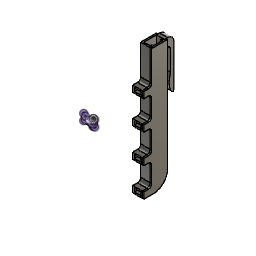
WaterLevelSensor (Autodesk Fusion 360 design; units mm, degrees)
Autodesk Fusion 360 part; units mm, degrees
note: some values were not read from the file. Set by a fixed rule: which sketch regions a step uses.
sketch "Sketch1" plane through (0, 0, 0) normal (1, 0, 0) x (0, 1, 0)
  line L0 (0, 200) -> (10, 200)
  line L1 (10, 200) -> (10, 129)
  line L2 (1, 120) -> (0, 120)
  line L3 (0, 120) -> (-5, 120)
  line L4 (-5, 120) -> (-5, 124)
  line L5 (-5, 124) -> (-2, 124)
  line L6 (-5, 142.3333) -> (-2, 142.3333)
  line L7 (-5, 138.3333) -> (-5, 142.3333)
  line L8 (-2, 138.3333) -> (-5, 138.3333)
  line L9 (-5, 160.6667) -> (-2, 160.6667)
  line L10 (-5, 156.6667) -> (-5, 160.6667)
  line L11 (-2, 156.6667) -> (-5, 156.6667)
  line L12 (-5, 179) -> (-2, 179)
  line L13 (-5, 175) -> (-5, 179)
  line L14 (-2, 175) -> (-5, 175)
  line L15 (0, 181) -> (0, 200)
  line L16 (0, 162.6667) -> (0, 173)
  line L17 (0, 126) -> (0, 136.3333)
  line L18 (0, 144.3333) -> (0, 154.6667)
  arc A0 (1, 120) -> (10, 129) centre (1, 129) ccw
  arc A1 (-2, 179) -> (0, 181) centre (-2, 181) ccw
  arc A2 (0, 173) -> (-2, 175) centre (-2, 173) ccw
  arc A3 (-2, 160.6667) -> (0, 162.6667) centre (-2, 162.6667) ccw
  arc A4 (0, 154.6667) -> (-2, 156.6667) centre (-2, 154.6667) ccw
  arc A5 (-2, 142.3333) -> (0, 144.3333) centre (-2, 144.3333) ccw
  arc A6 (0, 136.3333) -> (-2, 138.3333) centre (-2, 136.3333) ccw
  arc A7 (-2, 124) -> (0, 126) centre (-2, 126) ccw
  line L19 (0, 121) -> (-5, 121)
  line L20 (-5, 123) -> (-2, 123)
  arc A8 (-2, 123) -> (1, 126) centre (-2, 126) ccw
  line L21 (1, 126) -> (1, 136.3333)
  arc A9 (1, 136.3333) -> (-2, 139.3333) centre (-2, 136.3333) ccw
  line L22 (-2, 139.3333) -> (-5, 139.3333)
  line L23 (-5, 141.3333) -> (-2, 141.3333)
  arc A10 (-2, 141.3333) -> (1, 144.3333) centre (-2, 144.3333) ccw
  line L24 (1, 144.3333) -> (1, 154.6667)
  arc A11 (1, 154.6667) -> (-2, 157.6667) centre (-2, 154.6667) ccw
  line L25 (-2, 157.6667) -> (-5, 157.6667)
  line L26 (-5, 159.6667) -> (-2, 159.6667)
  arc A12 (-2, 159.6667) -> (1, 162.6667) centre (-2, 162.6667) ccw
  line L27 (1, 162.6667) -> (1, 173)
  arc A13 (1, 173) -> (-2, 176) centre (-2, 173) ccw
  line L28 (-2, 176) -> (-5, 176)
  line L29 (-5, 178) -> (-2, 178)
  arc A14 (-2, 178) -> (1, 181) centre (-2, 181) ccw
  line L30 (1, 181) -> (1, 200)
  line L31 (9, 200) -> (9, 129)
  arc A15 (1, 121) -> (9, 129) centre (1, 129) ccw
  line L32 (1, 121) -> (0, 121)
  line L33 (10, 200) -> (11, 200)
  line L34 (15, 196) -> (15, 170)
  line L35 (13, 180) -> (13, 193)
  line L36 (11, 195) -> (10, 195)
  spline S0 degree 5 poles (13, 180) (12.9242, 179.8) (12.7791, 179.4) (12.5813, 178.8) (12.3581, 178) (12.1509, 177) (12.0221, 176) (11.978, 175) (12.0221, 174) (12.1509, 173) (12.3581, 172) (12.5813, 171.2) (12.7791, 170.6) (12.9242, 170.2) (13, 170) knots 0 0 0 0 0 0 0.1 0.2 0.3 0.4 0.5 0.6 0.7 0.8 0.9 1 1 1 1 1 1
  arc A16 (15, 196) -> (11, 200) centre (11, 196) ccw
  arc A17 (13, 193) -> (11, 195) centre (11, 193) ccw
  spline S1 degree 5 poles (13, 170) (13.0376, 169.953) (13.1131, 169.8604) (13.227, 169.726) (13.38, 169.5556) (13.5735, 169.3586) (13.7694, 169.179) (13.9418, 169.0396) (14.076, 168.9434) (14.1707, 168.8813) (14.2252, 168.8475) (14.2391, 168.8391) knots 0 0 0 0 0 0 0.1 0.2 0.3 0.4 0.5 0.6 0.634052 0.634052 0.634052 0.634052 0.634052 0.634052
  line L37 (15, 170) -> (15, 169.2656)
  arc A18 (14.2391, 168.8391) -> (15, 169.2656) centre (14.5, 169.2656) ccw
  point P0 (0, 124)
  point P1 (12, 175)
  point P2 (14, 169)
  dimension "d1" = 10
  dimension "d2" = 80
  dimension "d3" = 5
  dimension "d4" = 4
  dimension "d10" = 9
  dimension "d11" = 2
  dimension "d12" = 4
  dimension "d13" = 2
  dimension "d14" = 0.5
  constraint horizontal L0
  constraint vertical L1
  constraint horizontal L2
  constraint vertical L17
  constraint horizontal L3
  constraint vertical L4
  constraint horizontal L5
  constraint collinear L15 L17
  constraint collinear L16 L17
  constraint collinear L17 L18
  constraint tangent L1 A0
  constraint tangent L2 A0
  constraint tangent L12 A1
  constraint tangent L15 A1
  constraint tangent L14 A2
  constraint tangent L16 A2
  constraint equal A1 A2
  constraint tangent L9 A3
  constraint tangent L16 A3
  constraint equal A1 A3
  constraint tangent L11 A4
  constraint tangent L18 A4
  constraint equal A1 A4
  constraint tangent L6 A5
  constraint tangent L18 A5
  constraint equal A1 A5
  constraint tangent L8 A6
  constraint tangent L17 A6
  constraint equal A1 A6
  constraint coincident P0 L5
  constraint coincident P0 L17
  constraint tangent L5 A7
  constraint tangent L17 A7
  constraint equal A1 A7
  constraint concentric A7 A8
  constraint concentric A6 A9
  constraint concentric A5 A10
  constraint concentric A4 A11
  constraint concentric A3 A12
  constraint concentric A2 A13
  constraint concentric A1 A14
  constraint concentric A0 A15
  constraint tangent L21 A9
  constraint tangent A9 L22
  constraint tangent A11 L25
  constraint tangent L20 A8
  constraint tangent L31 A15
  constraint tangent A8 L21
  constraint tangent L23 A10
  constraint tangent A10 L24
  constraint tangent L24 A11
  constraint tangent L27 A13
  constraint tangent L26 A12
  constraint tangent A12 L27
  constraint tangent A13 L28
  constraint tangent L29 A14
  constraint tangent A14 L30
  constraint tangent A15 L32
  constraint coincident L4 L20.start
  constraint coincident L4 L19.end
  constraint coincident L0 L31.start
  constraint coincident L0 L30.end
  constraint perpendicular L1 L33
  constraint perpendicular L33 L34
  constraint coincident L1 L36.end
  constraint perpendicular L1 L36
  constraint tangent L33 A16
  constraint tangent L34 A16
  constraint tangent L35 A17
  constraint tangent L36 A17
  constraint tangent S1 A18
  constraint tangent L37 A18
  measures "d1" distance of L0.start L0.end
  measures "d2" distance of L0.start L2.end
  measures "d3" distance of L2.end L3.end
  measures "d4" distance of L2.end P0
  measures "d10" radius of A0
  measures "d11" radius of A1
  measures "d12" radius of A16
  measures "d13" radius of A17
  measures "d14" radius of A18
extrude "Extrude1" add sketch "Sketch1" along normal blind 1 makes body 1
extrude "Extrude2" add sketch "Sketch1" along normal blind 6 contours L0 L12 L13 L15 A1 L29 A14 L30 | L0 L1 L2 L3 L4 A0 L19 L31 A15 L32 | L1 L33 L34 L35 L36 S0 A16 A17 S1 L37 A18 | L9 L10 L13 L14 L16 A2 A3 L26 A12 L27 A13 L28 | L4 L5 L7 L8 L17 A6 A7 L20 A8 L21 A9 L22 | L6 L7 L10 L11 L18 A4 A5 L23 A10 L24 A11 L25 bodies 1
extrude "Extrude3" cut sketch "Sketch1" along normal blind 1 contours L1 L33 L34 L35 L36 S0 A16 A17 S1 L37 A18 bodies 1
sketch "Sketch2" plane through (6, 0, 0) normal (1, 0, 0) x (0, 1, 0)
  spline S0 degree 5 poles (13, 180) (12.9242, 179.8) (12.7791, 179.4) (12.5813, 178.8) (12.3581, 178) (12.1509, 177) (12.0221, 176) (11.978, 175) (12.0221, 174) (12.1509, 173) (12.3581, 172) (12.5813, 171.2) (12.7791, 170.6) (12.9242, 170.2) (13, 170) knots 0 0 0 0 0 0 0.1 0.2 0.3 0.4 0.5 0.6 0.7 0.8 0.9 1 1 1 1 1 1
  spline S1 degree 5 poles (13, 170) (13.0376, 169.953) (13.1131, 169.8604) (13.227, 169.726) (13.38, 169.5556) (13.5735, 169.3586) (13.7694, 169.179) (13.9418, 169.0396) (14.076, 168.9434) (14.1707, 168.8813) (14.2252, 168.8475) (14.2391, 168.8391) knots 0 0 0 0 0 0 0.1 0.2 0.3 0.4 0.5 0.6 0.634052 0.634052 0.634052 0.634052 0.634052 0.634052
  arc A0 (14.2391, 168.8391) -> (15, 169.2656) centre (14.5, 169.2656) ccw
  line L0 (15, 169.2656) -> (15, 196)
  arc A1 (15, 196) -> (11, 200) centre (11, 196) ccw
  line L1 (11, 200) -> (9, 200)
  line L2 (9, 200) -> (9, 129)
  arc A2 (1, 121) -> (9, 129) centre (1, 129) ccw
  line L3 (1, 121) -> (-5, 121)
  line L4 (-5, 121) -> (-5, 120)
  line L5 (-5, 120) -> (1, 120)
  arc A3 (1, 120) -> (10, 129) centre (1, 129) ccw
  line L6 (10, 129) -> (10, 195)
  line L7 (10, 195) -> (11, 195)
  arc A4 (13, 193) -> (11, 195) centre (11, 193) ccw
  line L8 (13, 193) -> (13, 180)
  line L9 (-5, 178) -> (-2, 178)
  arc A5 (-2, 178) -> (1, 181) centre (-2, 181) ccw
  line L10 (1, 181) -> (1, 200)
  line L11 (1, 200) -> (0, 200)
  line L12 (0, 200) -> (0, 181)
  arc A6 (-2, 179) -> (0, 181) centre (-2, 181) ccw
  line L13 (-2, 179) -> (-5, 179)
  line L14 (-5, 179) -> (-5, 178)
  line L15 (-5, 159.6667) -> (-2, 159.6667)
  arc A7 (-2, 159.6667) -> (1, 162.6667) centre (-2, 162.6667) ccw
  line L16 (1, 162.6667) -> (1, 173)
  arc A8 (1, 173) -> (-2, 176) centre (-2, 173) ccw
  line L17 (-2, 176) -> (-5, 176)
  line L18 (-5, 176) -> (-5, 175)
  line L19 (-5, 175) -> (-2, 175)
  arc A9 (0, 173) -> (-2, 175) centre (-2, 173) ccw
  line L20 (0, 173) -> (0, 162.6667)
  arc A10 (-2, 160.6667) -> (0, 162.6667) centre (-2, 162.6667) ccw
  line L21 (-2, 160.6667) -> (-5, 160.6667)
  line L22 (-5, 160.6667) -> (-5, 159.6667)
  line L23 (-5, 141.3333) -> (-2, 141.3333)
  arc A11 (-2, 141.3333) -> (1, 144.3333) centre (-2, 144.3333) ccw
  line L24 (1, 144.3333) -> (1, 154.6667)
  arc A12 (1, 154.6667) -> (-2, 157.6667) centre (-2, 154.6667) ccw
  line L25 (-2, 157.6667) -> (-5, 157.6667)
  line L26 (-5, 157.6667) -> (-5, 156.6667)
  line L27 (-5, 156.6667) -> (-2, 156.6667)
  arc A13 (0, 154.6667) -> (-2, 156.6667) centre (-2, 154.6667) ccw
  line L28 (0, 154.6667) -> (0, 144.3333)
  arc A14 (-2, 142.3333) -> (0, 144.3333) centre (-2, 144.3333) ccw
  line L29 (-2, 142.3333) -> (-5, 142.3333)
  line L30 (-5, 142.3333) -> (-5, 141.3333)
  line L31 (-5, 123) -> (-2, 123)
  arc A15 (-2, 123) -> (1, 126) centre (-2, 126) ccw
  line L32 (1, 126) -> (1, 136.3333)
  arc A16 (1, 136.3333) -> (-2, 139.3333) centre (-2, 136.3333) ccw
  line L33 (-2, 139.3333) -> (-5, 139.3333)
  line L34 (-5, 139.3333) -> (-5, 138.3333)
  line L35 (-5, 138.3333) -> (-2, 138.3333)
  arc A17 (0, 136.3333) -> (-2, 138.3333) centre (-2, 136.3333) ccw
  line L36 (0, 136.3333) -> (0, 126)
  arc A18 (-2, 124) -> (0, 126) centre (-2, 126) ccw
  line L37 (-2, 124) -> (-5, 124)
  line L38 (-5, 124) -> (-5, 123)
  line L39 (-5, 139.3333) -> (-2, 139.3333)
  arc A19 (1, 136.3333) -> (-2, 139.3333) centre (-2, 136.3333) ccw
  line L40 (1, 136.3333) -> (1, 126)
  arc A20 (-2, 123) -> (1, 126) centre (-2, 126) ccw
  line L41 (-2, 123) -> (-5, 123)
  line L42 (-5, 123) -> (-5, 121)
  line L43 (-5, 121) -> (1, 121)
  arc A21 (1, 121) -> (9, 129) centre (1, 129) ccw
  line L44 (9, 129) -> (9, 200)
  line L45 (9, 200) -> (1, 200)
  line L46 (1, 200) -> (1, 181)
  arc A22 (-2, 178) -> (1, 181) centre (-2, 181) ccw
  line L47 (-2, 178) -> (-5, 178)
  line L48 (-5, 178) -> (-5, 176)
  line L49 (-5, 176) -> (-2, 176)
  arc A23 (1, 173) -> (-2, 176) centre (-2, 173) ccw
  line L50 (1, 173) -> (1, 162.6667)
  arc A24 (-2, 159.6667) -> (1, 162.6667) centre (-2, 162.6667) ccw
  line L51 (-2, 159.6667) -> (-5, 159.6667)
  line L52 (-5, 159.6667) -> (-5, 157.6667)
  line L53 (-5, 157.6667) -> (-2, 157.6667)
  arc A25 (1, 154.6667) -> (-2, 157.6667) centre (-2, 154.6667) ccw
  line L54 (1, 154.6667) -> (1, 144.3333)
  arc A26 (-2, 141.3333) -> (1, 144.3333) centre (-2, 144.3333) ccw
  line L55 (-2, 141.3333) -> (-5, 141.3333)
  line L56 (-5, 141.3333) -> (-5, 139.3333)
  line L57 (10, 195) -> (10, 200)
  line L58 (1.2, 200) -> (1.2, 181)
  arc A27 (-2, 177.8) -> (1.2, 181) centre (-2, 181) ccw
  line L59 (-2, 177.8) -> (-4.8, 177.8)
  line L60 (-4.8, 177.8) -> (-4.8, 176.2)
  line L61 (-4.8, 176.2) -> (-2, 176.2)
  arc A28 (1.2, 173) -> (-2, 176.2) centre (-2, 173) ccw
  line L62 (1.2, 173) -> (1.2, 162.6667)
  arc A29 (-2, 159.4667) -> (1.2, 162.6667) centre (-2, 162.6667) ccw
  line L63 (-2, 159.4667) -> (-4.8, 159.4667)
  line L64 (-4.8, 159.4667) -> (-4.8, 157.8667)
  line L65 (-4.8, 157.8667) -> (-2, 157.8667)
  arc A30 (1.2, 154.6667) -> (-2, 157.8667) centre (-2, 154.6667) ccw
  line L66 (1.2, 154.6667) -> (1.2, 144.3333)
  arc A31 (-2, 141.1333) -> (1.2, 144.3333) centre (-2, 144.3333) ccw
  line L67 (-2, 141.1333) -> (-4.8, 141.1333)
  line L68 (-4.8, 141.1333) -> (-4.8, 139.5333)
  line L69 (-4.8, 139.5333) -> (-2, 139.5333)
  arc A32 (1.2, 136.3333) -> (-2, 139.5333) centre (-2, 136.3333) ccw
  line L70 (1.2, 136.3333) -> (1.2, 126)
  arc A33 (-2, 122.8) -> (1.2, 126) centre (-2, 126) ccw
  line L71 (-2, 122.8) -> (-4.8, 122.8)
  line L72 (-4.8, 122.8) -> (-4.8, 121.2)
  line L73 (-4.8, 121.2) -> (1, 121.2)
  arc A34 (1, 121.2) -> (8.8, 129) centre (1, 129) ccw
  line L74 (8.8, 129) -> (8.8, 200)
  arc A35 (-0.7194, 177) -> (2.2, 181) centre (-2, 181) ccw
  line L75 (2.2, 200) -> (2.2, 181)
  line L76 (7.8, 129) -> (7.8, 200)
  arc A36 (1, 122.2) -> (7.8, 129) centre (1, 129) ccw
  line L77 (-0.2111, 122.2) -> (1, 122.2)
  arc A37 (-0.2111, 122.2) -> (2.2, 126) centre (-2, 126) ccw
  line L78 (2.2, 136.3333) -> (2.2, 126)
  arc A38 (2.2, 136.3333) -> (-0.7194, 140.3333) centre (-2, 136.3333) ccw
  arc A39 (-0.7194, 140.3333) -> (2.2, 144.3333) centre (-2, 144.3333) ccw
  line L79 (2.2, 154.6667) -> (2.2, 144.3333)
  arc A40 (2.2, 154.6667) -> (-0.7194, 158.6667) centre (-2, 154.6667) ccw
  arc A41 (-0.7194, 158.6667) -> (2.2, 162.6667) centre (-2, 162.6667) ccw
  line L80 (2.2, 173) -> (2.2, 162.6667)
  arc A42 (2.2, 173) -> (-0.7194, 177) centre (-2, 173) ccw
  constraint coincident L6.end L7.start
  constraint midpoint L1 L57.end
  constraint concentric A22 A27
  constraint concentric A23 A28
  constraint concentric A24 A29
  constraint concentric A25 A30
  constraint concentric A26 A31
  constraint concentric A19 A32
  constraint concentric A20 A33
  constraint concentric A21 A34
  constraint tangent L62 A29
  constraint tangent L61 A28
  constraint tangent A28 L62
  constraint tangent L58 A27
  constraint tangent A27 L59
  constraint tangent A29 L63
  constraint tangent L65 A30
  constraint tangent A30 L66
  constraint tangent L66 A31
  constraint tangent A31 L67
  constraint tangent L69 A32
  constraint tangent A32 L70
  constraint tangent L70 A33
  constraint tangent A33 L71
  constraint tangent L73 A34
  constraint tangent A34 L74
  constraint concentric A22 A35
  constraint concentric A21 A36
  constraint concentric A20 A37
  constraint concentric A19 A38
  constraint concentric A26 A39
  constraint concentric A25 A40
  constraint concentric A24 A41
  constraint concentric A23 A42
  constraint tangent L76 A36
  constraint tangent A37 L78
  constraint tangent A35 L75
  constraint tangent A36 L77
  constraint tangent L78 A38
  constraint tangent A39 L79
  constraint tangent L79 A40
  constraint tangent A41 L80
  constraint tangent L80 A42
extrude "Extrude4" add sketch "Sketch2" along normal blind 1 separate body contours L1 L2 A2 L3 L4 L5 A3 L6 L43 A21 L44 L57 | L2 A2 L3 L9 A5 L10 L15 A7 L16 A8 L17 L23 A11 L24 A12 L25 L31 A15 L32 A16 L33 L39 A19 L40 A20 L41 L42 L43 A21 L44 L45 L46 A22 L47 L48 L49 A23 L50 A24 L51 L52 L53 A25 L54 A26 L55 L56 L58 A27 L59 L60 L61 A28 L62 A29 L63 L64 L65 A30 L66 A31 L67 L68 L69 A32 L70 A33 L71 L72 L73 A34 L74 | L45 L58 A27 L59 L60 L61 A28 L62 A29 L63 L64 L65 A30 L66 A31 L67 L68 L69 A32 L70 A33 L71 L72 L73 A34 L74 A35 L75 L76 A36 L77 A37 L78 A38 A39 L79 A40 A41 L80 A42 | L45 A35 L75 L76 A36 L77 A37 L78 A38 A39 L79 A40 A41 L80 A42 | L31 A15 L32 A16 L33 L34 L35 A17 L36 A18 L37 L38 L39 A19 L40 A20 L41 | L9 A5 L10 L11 L12 A6 L13 L14 L46 A22 L47 | L23 A11 L24 A12 L25 L26 L27 A13 L28 A14 L29 L30 L53 A25 L54 A26 L55 | L15 A7 L16 A8 L17 L18 L19 A9 L20 A10 L21 L22 L49 A23 L50 A24 L51 makes body 2
extrude "Extrude5" add sketch "Sketch2" against normal blind 1 contours L45 L58 A27 L59 L60 L61 A28 L62 A29 L63 L64 L65 A30 L66 A31 L67 L68 L69 A32 L70 A33 L71 L72 L73 A34 L74 A35 L75 L76 A36 L77 A37 L78 A38 A39 L79 A40 A41 L80 A42 bodies 2
ref_plane "WorkPlane1" through (3, -36, 177) normal (0, -1, 0) x (0, 0, -1)
sketch "Sketch3" plane through (0, -36, 0) normal (0, -1, 0) x (-1, 0, 0)
  line L0 (0, -179) -> (0, -175)
  line L1 (0, -175) -> (-6, -175)
  line L2 (-6, -175) -> (-6, -176)
  line L3 (-6, -176) -> (-1, -176)
  line L4 (-1, -176) -> (-1, -178)
  line L5 (-1, -178) -> (-6, -178)
  line L6 (-6, -178) -> (-6, -179)
  line L7 (-6, -179) -> (0, -179)
  line L8 (-6, -179) -> (-6, -175)
  line L9 (-6, -175) -> (-7, -175)
  line L10 (-7, -175) -> (-7, -179)
  line L11 (-7, -179) -> (-6, -179)
  line L12 (-6, -176.2) -> (-6, -177.8)
  line L13 (-6, -177.8) -> (-5, -177.8)
  line L14 (-5, -177.8) -> (-5, -176.2)
  line L15 (-5, -176.2) -> (-6, -176.2)
  line L16 (-1.2, -176.2) -> (-1.2, -177.8)
  line L17 (-4.8, -177.8) -> (-4.8, -176.2)
  line L18 (-6.2, -179) -> (-6.2, -179.2)
  circle A0 centre (-3.5, -177) radius 1
  line L19 (-1.2, -177.8) -> (-2.9, -177.8)
  line L20 (-4.1, -177.8) -> (-4.8, -177.8)
  line L21 (-4.8, -176.2) -> (-4.1, -176.2)
  line L22 (-2.9, -176.2) -> (-1.2, -176.2)
  dimension "d30" = 2
  constraint coincident L11 L18.start
  constraint coincident A0 L19.end
  constraint coincident A0 L20.start
  constraint collinear L19 L20
  constraint coincident A0 L21.end
  constraint coincident A0 L22.start
  constraint collinear L21 L22
  measures "d30" diameter of A0
extrude "Extrude6" add sketch "Sketch3" along normal blind 1 separate body makes body 3
extrude "Extrude7" add sketch "Sketch3" against normal blind 1 contours L17 A0 L20 L21 | L16 A0 L19 L22 bodies 3
extrude "Extrude8" cut sketch "Sketch3" along normal blind 3.4 contours A0 bodies 3
